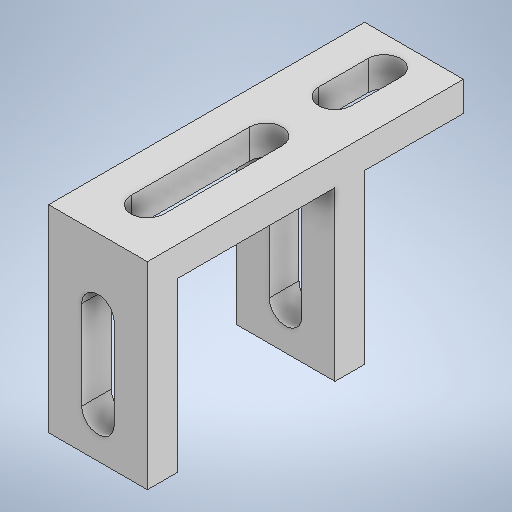
# Autodesk Inventor part: BeltMount1
Saved by Autodesk Inventor 2025.2 (Build 292293000, 293)
## iProperties
Created: 2025-07-28
Part Number: BeltMount1
Material: Generic
Document SubType Name: Modeling
Designer: Simon
Density: 1 g/cm^3
Appearance: Default
Author: Simon
Autodesk Inventor part; units mm, degrees
ref_plane "YZ Plane" through (0, 0, 0) normal (1, 0, 0) x (0, 1, 0)
ref_plane "XZ Plane" through (0, 0, 0) normal (0, 1, 0) x (-1, 0, 0)
ref_plane "XY Plane" through (0, 0, 0) normal (0, 0, 1) x (1, 0, 0)
sketch "Sketch1" plane through (0, 0, 0) normal (1, 0, 0) x (0, 1, 0)
  line L0 (-10, 11) -> (10, 11)
  line L1 (10, 11) -> (10, -11)
  line L2 (10, -11) -> (-10, -11)
  line L3 (-10, -11) -> (-10, 11)
  line L4 (-10, 11) -> (10, -11) construction
  line L5 (10, 11) -> (-10, -11) construction
  line L6 (-7, 8) -> (7, 8)
  line L7 (7, 8) -> (7, -8)
  line L8 (7, -8) -> (-7, -8)
  line L9 (-7, -8) -> (-7, 8)
  line L10 (-7, 8) -> (7, -8) construction
  line L11 (7, 8) -> (-7, -8) construction
  line L12 (-7, 8) -> (-10, 8)
  line L13 (-10, 8) -> (-10, -8)
  line L14 (-10, -8) -> (-7, -8)
  line L15 (-7, -8) -> (-7, 8)
  line L16 (10, -11) -> (7, -11)
  line L17 (7, -11) -> (7, -21)
  line L18 (7, -21) -> (10, -21)
  line L19 (10, -21) -> (10, -11)
  point P0 (0, 0)
  point P1 (7, -11)
  dimension "d0" = 20
  dimension "d1" = 22
  dimension "d2" = 14
  dimension "d3" = 16
  dimension "d4" = 3
  dimension "d5" = 10
  constraints: 40 end point, 8 parallel, 4 horizontal, 4 midpoint, 4 perpendicular, 1 point on line
  measures "d0" distance of L1.end L2.end
  measures "d1" distance of L0.end L1.end
  measures "d2" distance of L7.end L8.end
  measures "d3" distance of L6.end L7.end
  measures "d4" distance of L18.end L17.end
  measures "d5" distance of L17.end L16.end
extrude "Extrusion1" add sketch "Sketch1" along normal blind 10 contours L0 L1 L2 L3 L14 L8 L7 L6 L12 | L19 L18 L17 L2
sketch "Sketch2" plane through (0, 7, -8) normal (0, -1, 0) x (1, 0, 0)
  line L0 (10, 19) -> (10, 16) projected
  line L1 (0, 0) -> (0, -3) projected
  line L2 (10, 16) -> (0, 16)
  line L3 (0, 16) -> (0, 0)
  line L4 (0, 0) -> (10, 0)
  line L5 (10, 0) -> (10, 16)
  line L6 (5, 16) -> (5, 14)
  line L7 (5, 0) -> (5, 2)
  line L8 (5, 14) -> (5, 2) construction
  line L9 (3.35, 14) -> (3.35, 2)
  line L10 (6.65, 2) -> (6.65, 14)
  arc A0 (6.65, 14) -> (3.35, 14) centre (5, 14) ccw
  arc A1 (3.35, 2) -> (6.65, 2) centre (5, 2) ccw
  line L11 (0, -3) -> (0, -13) projected
  line L12 (10, -13) -> (0, -13)
  line L13 (0, -13) -> (0, -3)
  line L14 (0, -3) -> (10, -3)
  line L15 (10, -3) -> (10, -13)
  line L16 (5, -3) -> (5, -5)
  line L17 (5, -13) -> (5, -10)
  line L18 (5, -5) -> (5, -10) construction
  line L19 (3.35, -5) -> (3.35, -10)
  line L20 (6.65, -10) -> (6.65, -5)
  arc A2 (6.65, -5) -> (3.35, -5) centre (5, -5) ccw
  arc A3 (3.35, -10) -> (6.65, -10) centre (5, -10) ccw
  point P0 (0, 8)
  point P1 (5, 8)
  point P2 (5, -7.5)
  dimension "d8" = 2
  dimension "d9" = 2
  dimension "d10" = 3.3
  dimension "d11" = 2
  dimension "d12" = 3
  dimension "d13" = 3.3
  constraints: 40 end point, 8 point on circle, 8 tangent, 6 midpoint, 6 parallel, 6 vertical, 4 centre point, 2 horizontal, 2 perpendicular
  measures "d8" distance of L6.start L6.end
  measures "d9" distance of L7.start L7.end
  measures "d10" diameter of A1
  measures "d11" distance of L16.start L16.end
  measures "d12" distance of L17.start L17.end
  measures "d13" diameter of A3
extrude "Extrusion2" cut sketch "Sketch2" against normal through all contours A0 L10 A1 L9 | A2 L20 A3 L19
sketch "Sketch3" plane through (0, -10, 11) normal (0, 0, 1) x (1, 0, 0)
  line L0 (0, 0) -> (10, 0) projected
  line L1 (0, 17) -> (10, 17) projected
  line L2 (0, 0) -> (10, 0)
  line L3 (10, 0) -> (10, 17)
  line L4 (10, 17) -> (0, 17)
  line L5 (0, 17) -> (0, 0)
  line L6 (5, 17) -> (5, 13)
  line L7 (5, 0) -> (5, 4)
  line L8 (5, 13) -> (5, 4) construction
  line L9 (3.35, 13) -> (3.35, 4)
  line L10 (6.65, 4) -> (6.65, 13)
  arc A0 (6.65, 13) -> (3.35, 13) centre (5, 13) ccw
  arc A1 (3.35, 4) -> (6.65, 4) centre (5, 4) ccw
  point P0 (0, 10)
  point P1 (5, 8.5)
  dimension "d16" = 4
  dimension "d17" = 4
  dimension "d18" = 3.3
  constraints: 20 end point, 4 point on circle, 4 tangent, 3 midpoint, 3 parallel, 3 vertical, 2 centre point, 1 horizontal, 1 perpendicular
  measures "d16" distance of L6.start L6.end
  measures "d17" distance of L7.start L7.end
  measures "d18" diameter of A1
extrude "Extrusion3" cut sketch "Sketch3" against normal through all contours A1 L9 A0 L10
body "Solid1"
